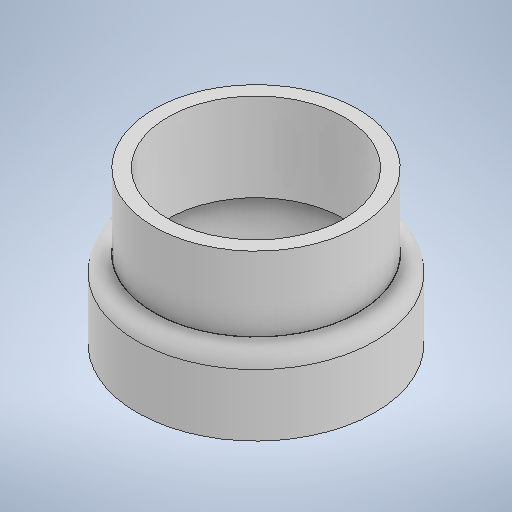
# Autodesk Inventor part: Male Adaptor to Water Sensor
Saved by Autodesk Inventor 2025 (Build 290162000, 162)
## iProperties
Created: 2024-07-09
Part Number: Male Adaptor to Water Sensor
Material: Generic
Document SubType Name: Modeling
Designer: track
Density: 1 g/cm^3
Appearance: Default
Author: track
Autodesk Inventor part; units mm, degrees
ref_plane "YZ Plane" through (0, 0, 0) normal (1, 0, 0) x (0, 1, 0)
ref_plane "XZ Plane" through (0, 0, 0) normal (0, 1, 0) x (-1, 0, 0)
ref_plane "XY Plane" through (0, 0, 0) normal (0, 0, 1) x (1, 0, 0)
sketch "Sketch1" plane through (0, 0, 0) normal (0, 0, 1) x (1, 0, 0)
  line L0 (0, 0) -> (0, 29.5332)
  line L1 (29.4, 44) -> (29.4, 22.6)
  line L2 (29.4, 22.6) -> (29.4875, 22.6)
  line L3 (34.25, 17.8375) -> (34.25, 0)
  line L4 (34.25, 0) -> (30.25, 0)
  line L5 (25.4, 44) -> (29.4, 44)
  line L6 (25.4, 44) -> (25.4, 18.6)
  line L7 (25.4, 18.6) -> (30.25, 18.6)
  line L8 (30.25, 18.6) -> (30.25, 0)
  arc A0 (34.25, 17.8375) -> (29.4875, 22.6) centre (29.4875, 17.8375) ccw
  dimension "d0" = 25.4
  dimension "d1" = 30.25
  dimension "d2" = 4
  dimension "d3" = 4
  dimension "d4" = 25.4
  dimension "d5" = 44
  dimension "d6" = 0
  dimension "d7" = 4
  dimension "d8" = 4.7625
  constraints: 19 end point, 5 perpendicular, 2 horizontal, 2 point on circle, 2 tangent, 2 vertical, 1 centre point
  measures "d0" distance between parallel lines of L0 L6
  measures "d1" distance between parallel lines of L0 L8
  measures "d2" distance between parallel lines of L8 L3
  measures "d3" distance between parallel lines of L6 L1
  measures "d4" distance between parallel lines of L7 L5
  measures "d5" distance between parallel lines of L4 L5
  measures "d6" distance from line of L0.start L4
  measures "d7" distance between parallel lines of L7 L2
  measures "d8" radius of A0
revolve "Revolution1" add sketch "Sketch1" angle 360 about axis through (0, 0, 0) along (0, 1, 0)
body "Solid1"
